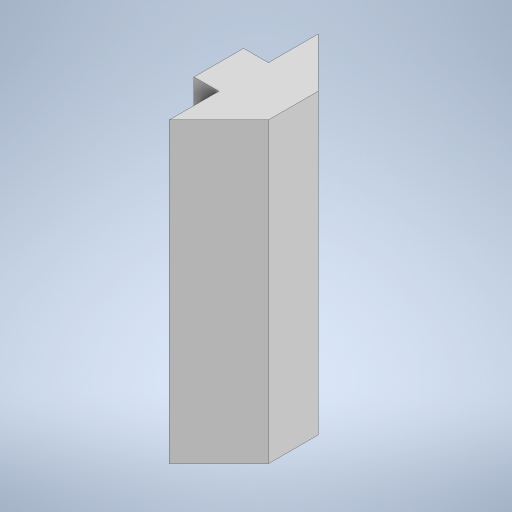
# Autodesk Inventor part: Dyenhtyytt cjtlbytybt
Saved by Autodesk Inventor 2023 (Build 270158000, 158)
## iProperties
Created: 2022-05-06
Part Number: Dyenhtyytt cjtlbytybt
Material: Типовые
Document SubType Name: Modeling
Designer: avkap
Density: 1 g/cm^3
Appearance: По умолчанию
Author: avkap
Autodesk Inventor part; units mm, degrees
ref_plane "YZ Plane" through (0, 0, 0) normal (1, 0, 0) x (0, 1, 0)
ref_plane "XZ Plane" through (0, 0, 0) normal (0, 1, 0) x (-1, 0, 0)
ref_plane "XY Plane" through (0, 0, 0) normal (0, 0, 1) x (1, 0, 0)
sketch "Эскиз1" plane through (0, 0, 0) normal (0, 1, 0) x (-1, 0, 0)
  line L0 (0, 0) -> (0, -10)
  line L1 (0, -10) -> (-5, -10)
  line L2 (-5, -10) -> (-5, -20)
  line L3 (-5, -20) -> (-5, 0)
  line L4 (-5, 0) -> (0, 0)
  line L5 (-5, 0) -> (-5, 10)
  line L6 (-5, 0) -> (-15, 0)
  line L7 (-15, 0) -> (-5, 10)
  line L8 (-15, 0) -> (-15, -10)
  line L9 (-15, -10) -> (-5, -20)
  dimension "d2" = 10
  dimension "d3" = 5
  dimension "d4" = 10
  dimension "d5" = 10
  dimension "d6" = 10
  constraints: 20 end point, 4 perpendicular, 4 point on line, 1 vertical
  measures "d2" distance of L0.start L0.end
  measures "d3" distance of L0.end L1.end
  measures "d4" distance of L1.end L2.end
  measures "d5" distance of L3.end L5.end
  measures "d6" distance of L3.end L6.end
extrude "Выдавливание1" add sketch "Эскиз1" along normal blind 60
